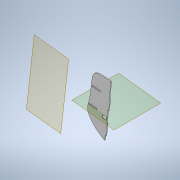
# Autodesk Inventor part: поперечная_поддержка
Saved by Autodesk Inventor 2020 (Build 240168000, 168)
## iProperties
Created: 2022-03-08
Part Number: поперечная_поддержка
Material: Типовые
Document SubType Name: Modeling
Designer: Администратор
Density: 1 g/cm^3
Appearance: По умолчанию
Author: Администратор
Autodesk Inventor part; units mm, degrees
ref_plane "YZ Plane" through (0, 0, 0) normal (1, 0, 0) x (0, 1, 0)
ref_plane "XZ Plane" through (0, 0, 0) normal (0, 1, 0) x (-1, 0, 0)
ref_plane "XY Plane" through (0, 0, 0) normal (0, 0, 1) x (1, 0, 0)
ref_plane "РабПлоскость1" through (-276.9669, -64.4178, 0) normal (0, 0, 1) x (0.9934395, -0.1143588, 0)
sketch "Эскиз1" plane through (-276.9669, -64.4178, 0) normal (0, 0, 1) x (0.9934395, -0.1143588, 0)
  line L0 (291.0502, 248.6307) -> (221.0654, 248.6307) construction
  line L1 (221.0654, 248.6307) -> (209.9068, 234.7693) construction
  line L2 (209.9068, 234.7693) -> (196.6601, 234.7693) construction
  line L3 (196.6601, 234.7693) -> (196.6601, 175.7756) construction
  line L4 (196.6601, 175.7756) -> (196.6601, 136.8397) construction
  line L5 (196.6601, 136.8397) -> (196.6601, 100.2635) construction
  line L6 (196.6601, 100.2635) -> (185.4513, 58.9679) construction
  line L7 (185.4513, 58.9679) -> (192.5305, 32.4207) construction
  line L8 (192.5305, 32.4207) -> (238.9418, -16.2312) construction
  line L9 (238.9418, -16.2312) -> (291.0502, -35.7278) construction
  spline S0 degree 4 poles (291.0502, 248.6307) (221.0654, 248.6307) (209.9068, 234.7693) (196.6601, 234.7693) (196.6601, 175.7756) (196.6601, 136.8397) (196.6601, 100.2635) (185.4513, 58.9679) (192.5305, 32.4207) (238.9418, -16.2312) (291.0502, -35.7278) knots 1 1 1 1 1 2 3 4 5 6 7 8 8 8 8 8
  line L10 (291.0502, 248.6307) -> (291.0502, -35.7278)
  line L11 (295.0502, 248.6307) -> (291.0502, 248.6307) projected
  line L12 (291.0502, 248.6307) -> (591.0502, 248.6307) construction
  line L13 (291.0502, 248.6307) -> (-95.7817, 248.6307)
  line L14 (295.0502, -35.7278) -> (291.0502, -35.7278) projected
  line L15 (291.0502, -35.7278) -> (207.0762, -35.7278)
  point P0 (267.7832, 95.6688)
  constraints: 8 end point, 4 horizontal, 4 vertical, 1 point on line, 3 other
extrude "Выдавливание1" add sketch "Эскиз1" along normal mid plane 4
sketch "Эскиз2" plane through (10.9482, -108.3491, 1.5) normal (0.9934395, -0.1143588, 0) x (0, 0, -1)
  line L0 (3, 0) -> (0, 0) projected
  line L1 (0, 0) -> (0, 59.7017)
  line L2 (-0.5, -25.0103) -> (-0.5, 259.3482) projected
  line L3 (3.5, 259.3482) -> (3.5, -25.0103) projected
  line L4 (3, 59.7017) -> (3, 119.4034)
  line L5 (0, 119.4034) -> (0, 179.1051)
  line L6 (0, 179.1051) -> (3, 179.1051)
  line L7 (3, 179.1051) -> (3, 238.8068)
  line L8 (0, 238.8068) -> (0, 298.5085)
  line L9 (0, 298.5085) -> (3, 298.5085) projected
  line L10 (0, 59.7017) -> (3, 59.7017)
  line L11 (3, 119.4034) -> (0, 119.4034)
  line L12 (3, 238.8068) -> (0, 238.8068)
  line L13 (0, 59.7017) -> (0, 119.4034)
  line L14 (0, 179.1051) -> (0, 238.8068)
  line L15 (3, 238.8068) -> (3, 298.5085)
  line L16 (0, 298.5085) -> (3, 298.5085)
  line L17 (0, 0) -> (3, 0)
  line L18 (3, 59.7017) -> (3, 0)
  line L19 (3, 59.7017) -> (0, 59.7017)
  line L20 (0, 119.4034) -> (3, 119.4034)
  line L21 (0, 59.7017) -> (0, 119.4034)
  line L22 (3, 179.1051) -> (0, 179.1051)
  line L23 (0, 238.8068) -> (3, 238.8068)
  line L24 (3, 238.8068) -> (3, 298.5085)
  line L25 (0, 298.5085) -> (3, 298.5085)
  line L26 (0, 238.8068) -> (0, 298.5085)
  line L27 (3, 179.1051) -> (3.5, 179.1051)
  line L28 (3, 119.4034) -> (3.5, 119.4034)
  line L29 (3.5, 179.1051) -> (3.5, 119.4034)
  line L30 (0, 179.1051) -> (-0.5, 179.1051)
  line L31 (-0.5, 179.1051) -> (-0.5, 119.4034)
  line L32 (0, 119.4034) -> (-0.5, 119.4034)
  line L33 (3, 59.7017) -> (3.5, 59.7017)
  line L34 (3.5, 59.7017) -> (3.5, 0)
  line L35 (3, 0) -> (3.5, 0)
  line L36 (0, 0) -> (-0.5, 0)
  line L37 (-0.5, 0) -> (-0.5, 59.7017)
  line L38 (-0.5, 59.7017) -> (0, 59.7017)
  point P0 (1.5, 106.3863)
  point P1 (3.5, -25.0103)
  point P2 (3, 59.7017)
  constraints: 68 end point, 9 point on line, 7 perpendicular, 7 vertical, 6 horizontal, 4 parallel, 3 collinear, 18 other
extrude "Выдавливание2" add sketch "Эскиз2" along normal blind 4 contours L0 L1 L10 L18 | L18 L33 L3 L35 | L36 L2 L38 L1 | L11 L5 L6 L27 L3 L28 | L32 L2 L30 L5
sketch "Эскиз3" plane through (-276.9669, -64.4178, 0) normal (0, 0, 1) x (0.9934395, -0.1143588, 0)
  point P0 (267.7832, 95.6688)
sketch "Эскиз4" plane through (-276.9669, -64.4178, 0) normal (0, 0, 1) x (0.9934395, -0.1143588, 0)
  line L0 (-21.9452, -13.2655) -> (34.011, -13.2655) projected
  line L1 (-21.9452, -13.2655) -> (34.011, -13.2655) projected
  line L2 (34.011, -13.2655) -> (34.011, -16.2655) projected
  line L3 (-21.9452, -13.2655) -> (34.011, -13.2655) projected
  line L4 (-21.9452, -16.2655) -> (-21.9452, -13.2655) projected
  line L5 (34.011, -16.2655) -> (-21.9452, -16.2655) projected
  line L6 (-21.9452, -16.2655) -> (-21.9452, -13.2655)
  line L7 (-69.5874, -16.2655) -> (-21.9452, -16.2655)
  line L8 (-21.9452, -13.2655) -> (-69.5874, -13.2655)
  line L9 (-69.5874, -13.2655) -> (-69.5874, -16.2655)
  line L10 (-21.9452, -13.2655) -> (-21.9452, -12.7655)
  line L11 (-21.9452, -12.7655) -> (-69.5874, -12.7655)
  line L12 (-69.5874, -12.7655) -> (-69.5874, -13.2655)
  line L13 (-69.5874, -16.2655) -> (-69.5874, -16.7655)
  line L14 (-69.5874, -16.7655) -> (-21.9452, -16.7655)
  line L15 (-21.9452, -16.7655) -> (-21.9452, -16.2655)
  point P0 (267.7832, 95.6688)
  point P1 (-66.0194, -13.2655)
  dimension "d16" = 0.5
  dimension "d17" = 0.5
  constraints: 20 end point, 4 perpendicular, 3 point on line, 2 collinear, 1 coincident, 1 horizontal, 1 parallel, 1 vertical
  measures "d16" distance of L0.start L10.end
  measures "d17" distance of L7.start L13.end
extrude "Выдавливание3" cut sketch "Эскиз4" against normal through all both and the other way through all contours L4 L7 L9 L8 | L8 L12 L11 L10 | L15 L14 L13 L7
sketch "Эскиз5" plane through (-276.9669, -64.4178, 0) normal (0, 0, 1) x (0.9934395, -0.1143588, 0)
  line L0 (291.0502, 173.347) -> (291.0502, 169.347) projected
  line L1 (246.0502, 173.347) -> (291.0502, 173.347) projected
  line L2 (246.0502, 173.347) -> (246.0502, 169.347) projected
  line L3 (291.0502, 169.347) -> (246.0502, 169.347) projected
  line L4 (246.0502, 173.347) -> (246.0502, 169.347)
  line L5 (186.6761, 173.347) -> (246.0502, 173.347)
  line L6 (186.6761, 173.347) -> (186.6761, 169.347)
  line L7 (186.6761, 169.347) -> (246.0502, 169.347)
  line L8 (246.0502, 173.347) -> (246.0502, 169.347)
  line L9 (186.6761, 173.347) -> (186.6761, 173.847)
  line L10 (186.6761, 173.847) -> (246.0502, 173.847)
  line L11 (246.0502, 173.847) -> (246.0502, 173.347)
  line L12 (246.0502, 169.347) -> (246.0502, 168.847)
  line L13 (246.0502, 168.847) -> (186.6761, 168.847)
  line L14 (186.6761, 168.847) -> (186.6761, 169.347)
  point P0 (267.7832, 95.6688)
  dimension "d14" = 0.5
  dimension "d15" = 0.5
  constraints: 22 end point, 4 perpendicular, 4 vertical, 2 collinear, 1 parallel
  measures "d14" distance of L5.start L9.end
  measures "d15" distance of L2.end L12.end
sketch "Эскиз6" plane through (-276.9669, -64.4178, -2) normal (0, 0, -1) x (-0.9934395, 0.1143588, 0)
  line L0 (16.8024, -31.0891) -> (36.8024, -31.0891)
  line L1 (36.8024, -31.0891) -> (36.8024, -46.0891)
  line L2 (36.8024, -46.0891) -> (16.8024, -46.0891)
  line L3 (16.8024, -46.0891) -> (16.8024, -31.0891)
  line L4 (-286.6513, 74.0401) -> (-286.6513, 59.0401)
  line L5 (-286.6513, 59.0401) -> (-266.6513, 59.0401)
  line L6 (-266.6513, 59.0401) -> (-266.6513, 74.0401)
  line L7 (-266.6513, 74.0401) -> (-286.6513, 74.0401)
  point P0 (-267.7832, 95.6688)
  dimension "d10" = 20
  dimension "d11" = 15
  dimension "d18" = 15
  dimension "d19" = 20
  constraints: 16 end point, 6 perpendicular, 1 horizontal, 1 vertical
  measures "d10" distance of L0.start L0.end
  measures "d11" distance of L0.end L1.end
  measures "d18" distance of L4.start L4.end
  measures "d19" distance of L4.end L5.end
extrude "Выдавливание6" cut sketch "Эскиз6" against normal through all contours L7 L6 L5 L4
ref_plane "РабПлоскость2" through (1.8532, -16.6155, -86.2852) normal (-0.1143588, -0.9934395, 0) x (0, 0, 1)
sketch "Эскиз8" plane through (1.8532, -16.6155, -86.2852) normal (-0.1143588, -0.9934395, 0) x (0, 0, 1)
  line L0 (88.2852, 35.4303) -> (84.2852, 35.4303) projected
  line L1 (84.2852, 35.4303) -> (84.2852, 89.0995)
  line L2 (84.2852, 89.0995) -> (88.2852, 89.0995)
  line L3 (88.2852, 89.0995) -> (88.2852, 35.4303)
  point P0 (86.2852, 3.7412)
  constraints: 6 end point, 2 perpendicular, 1 vertical
extrude "Выдавливание7" cut sketch "Эскиз8" along normal blind 1 and the other way blind 3
extrude "Выдавливание8" cut sketch "Эскиз5" against normal through all both and the other way through all contours L2 L7 L6 L5
